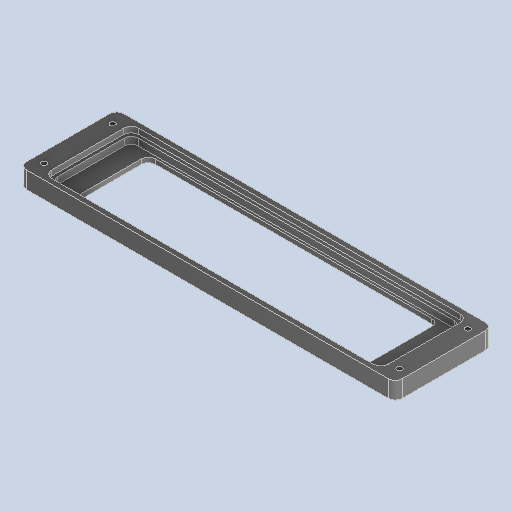
# Autodesk Inventor part: TorsoButtonCoverFrame
Saved by Autodesk Inventor 2024.2 (Build 282272000, 272)
## iProperties
Created: 2024-01-28
Part Number: TorsoButtonCoverFrame
Material: Acetal Resin, Black
Document SubType Name: Modeling
Designer: Masato Kubotera
Density: 1.425 g/cm^3
Appearance: Smooth - Black
Vendor: meviy
Mass: 8.31049 g
Surface Area: 66.1312 cm^2
Volume: 5.83192 cm^3
Author: Masato Kubotera
Autodesk Inventor part; units mm, degrees
ref_plane "YZ Plane" through (0, 0, 0) normal (1, 0, 0) x (0, 1, 0)
ref_plane "XZ Plane" through (0, 0, 0) normal (0, 1, 0) x (-1, 0, 0)
ref_plane "XY Plane" through (0, 0, 0) normal (0, 0, 1) x (1, 0, 0)
derived "TorsoUpperFrame.ipt"
sketch "Sketch1" plane through (0, 0, 0) normal (0, 0, 1) x (1, 0, 0)
  line L0 (-50, -90) -> (50, -90)
  line L1 (50, -90) -> (50, 90)
  line L2 (50, 90) -> (-50, 90)
  line L3 (-50, 90) -> (-50, -90)
  line L4 (-50, -90) -> (50, 90) construction
  line L5 (50, -90) -> (-50, 90) construction
  line L6 (-50, 0) -> (50, 0)
  line L7 (0, -90) -> (0, 90) construction
  circle A0 centre (0, 0) radius 18.75
  line L8 (-12, -16) -> (31, -16) construction
  line L9 (31, -16) -> (31, 16) construction
  line L10 (31, 16) -> (-12, 16) construction
  line L11 (-12, 16) -> (-12, -16) construction
  line L12 (-12, -16) -> (31, 16) construction
  line L13 (31, -16) -> (-12, 16) construction
  line L14 (1, -13.5) -> (28, -13.5) construction
  line L15 (28, -13.5) -> (28, 13.5) construction
  line L16 (28, 13.5) -> (1, 13.5) construction
  line L17 (1, 13.5) -> (1, -13.5) construction
  line L18 (1, -13.5) -> (28, 13.5) construction
  line L19 (28, -13.5) -> (1, 13.5) construction
  line L20 (9.61, -16.1) -> (31.1, -16.1)
  line L21 (31.1, -16.1) -> (31.1, 16.1)
  line L22 (31.1, 16.1) -> (9.61, 16.1)
  line L23 (50, 85) -> (38, 85)
  line L24 (38, 85) -> (38, 90)
  line L25 (-15, 90) -> (-15, 85)
  line L26 (-15, 85) -> (15, 85)
  line L27 (15, 85) -> (15, 90)
  arc A1 (38, 85) -> (42, 85) centre (40, 85) ccw
  arc A2 (11, 85) -> (15, 85) centre (13, 85) ccw
  arc A3 (-15, 85) -> (-11, 85) centre (-13, 85) ccw
  line L28 (-38, 85) -> (-38, 90)
  arc A4 (-42, 85) -> (-38, 85) centre (-40, 85) ccw
  line L29 (-50, 85) -> (-38, 85)
  line L30 (46, 85) -> (46, 79) construction
  line L31 (-46, 85) -> (-46, 79) construction
  circle A5 centre (0, 0) radius 29 construction
  line L32 (-41.5, 0) -> (-41.5, 53.2624)
  line L33 (-41.5, 53.2624) -> (-50, 58.1699)
  circle A6 centre (-42.5, 62.5) radius 7.5 construction
  circle A7 centre (-42.5, 62.5) radius 5 construction
  line L34 (-70, -90.6743) -> (-70, 90) construction
  line L35 (70, -90.6743) -> (70, 90) construction
  line L36 (-50, 62.5) -> (-37.5, 62.5) construction
  circle A8 centre (-42.5, -62.5) radius 5 construction
  circle A9 centre (-42.5, -62.5) radius 7.5 construction
  line L37 (-41.5, 0) -> (-41.5, -53.2624)
  line L38 (-41.5, -53.2624) -> (-50, -58.1699)
  line L39 (-50, -85) -> (-38, -85)
  line L40 (-38, -85) -> (-38, -90)
  arc A10 (-38, -85) -> (-42, -85) centre (-40, -85) ccw
  line L41 (-15, -85) -> (15, -85)
  arc A11 (-11, -85) -> (-15, -85) centre (-13, -85) ccw
  arc A12 (15, -85) -> (11, -85) centre (13, -85) ccw
  line L42 (-15, -90) -> (-15, -85)
  line L43 (15, -85) -> (15, -90)
  arc A13 (42, -85) -> (38, -85) centre (40, -85) ccw
  line L44 (38, -85) -> (38, -90)
  line L45 (50, -85) -> (38, -85)
  line L46 (-36.6858, 30.1642) -> (-36.6858, 46.0358)
  line L47 (-34.6858, 48.0358) -> (-18.8142, 48.0358)
  line L48 (-35.6, 46.95) -> (-35.6, 29.25) construction
  line L49 (-17.9, 46.95) -> (-35.6, 46.95) construction
  line L50 (-36.1, 28.75) -> (-36.1, 47.45) construction
  line L51 (-36.1, 47.45) -> (-17.4, 47.45) construction
  line L52 (-35.6, 29.25) -> (-17.9, 29.25) construction
  line L53 (-35.6, 46.95) -> (-17.9, 29.25) construction
  line L54 (-17.9, 46.95) -> (-35.6, 29.25) construction
  line L55 (-18.8142, 28.1642) -> (-34.6858, 28.1642)
  line L56 (-16.8142, 48.0358) -> (-36.6858, 28.1642) construction
  line L57 (-36.6858, 48.0358) -> (-16.8142, 28.1642) construction
  line L58 (-17.4, 28.75) -> (-36.1, 28.75) construction
  line L59 (-36.1, 47.45) -> (-17.4, 28.75) construction
  line L60 (-17.4, 47.45) -> (-36.1, 28.75) construction
  line L61 (-17.9, 29.25) -> (-17.9, 46.95) construction
  line L62 (-17.4, 47.45) -> (-17.4, 28.75) construction
  arc A14 (-18.8142, 28.1642) -> (-16.8142, 30.1642) centre (-18.8142, 30.1642) ccw
  line L63 (-16.8142, 46.0358) -> (-16.8142, 30.1642)
  arc A15 (-36.6858, 30.1642) -> (-34.6858, 28.1642) centre (-34.6858, 30.1642) ccw
  arc A16 (-16.8142, 46.0358) -> (-18.8142, 48.0358) centre (-18.8142, 46.0358) ccw
  arc A17 (-34.6858, 48.0358) -> (-36.6858, 46.0358) centre (-34.6858, 46.0358) ccw
  arc A18 (-18.8142, -48.0358) -> (-16.8142, -46.0358) centre (-18.8142, -46.0358) ccw
  line L64 (-16.8142, -46.0358) -> (-16.8142, -30.1642)
  line L65 (-17.9, -29.25) -> (-17.9, -46.95) construction
  line L66 (-17.4, -47.45) -> (-17.4, -28.75) construction
  arc A19 (-16.8142, -30.1642) -> (-18.8142, -28.1642) centre (-18.8142, -30.1642) ccw
  line L67 (-34.6858, -48.0358) -> (-18.8142, -48.0358)
  line L68 (-17.9, -46.95) -> (-35.6, -46.95) construction
  line L69 (-36.1, -47.45) -> (-17.4, -47.45) construction
  line L70 (-18.8142, -28.1642) -> (-34.6858, -28.1642)
  line L71 (-35.6, -29.25) -> (-17.9, -29.25) construction
  line L72 (-35.6, -46.95) -> (-17.9, -29.25) construction
  line L73 (-17.9, -46.95) -> (-35.6, -29.25) construction
  line L74 (-17.4, -28.75) -> (-36.1, -28.75) construction
  line L75 (-36.1, -47.45) -> (-17.4, -28.75) construction
  line L76 (-17.4, -47.45) -> (-36.1, -28.75) construction
  line L77 (-16.8142, -48.0358) -> (-36.6858, -28.1642) construction
  line L78 (-36.6858, -48.0358) -> (-16.8142, -28.1642) construction
  arc A20 (-36.6858, -46.0358) -> (-34.6858, -48.0358) centre (-34.6858, -46.0358) ccw
  line L79 (-36.6858, -30.1642) -> (-36.6858, -46.0358)
  line L80 (-35.6, -46.95) -> (-35.6, -29.25) construction
  line L81 (-36.1, -28.75) -> (-36.1, -47.45) construction
  arc A21 (-34.6858, -28.1642) -> (-36.6858, -30.1642) centre (-34.6858, -30.1642) ccw
  arc A22 (0, 16) -> (-12, 10.583) centre (0, 0) ccw construction
  arc A23 (-12, -10.583) -> (0, -16) centre (0, 0) ccw construction
  line L82 (-26.75, 38.1) -> (-26.75, -38.1) construction
  line L83 (-14.5, 55) -> (-27.6628, 55)
  arc A24 (-39.3295, 80) -> (-41.0778, 77.0287) centre (-39.3295, 78) ccw
  line L84 (-41.5, 16) -> (-37.5, 16) construction
  line L85 (-41.5, -16) -> (-37.5, -16) construction
  line L86 (-37.25, -49) -> (-16.25, -49) construction
  line L87 (-14.25, -47) -> (-14.25, 47) construction
  line L88 (-16.25, 49) -> (-37.25, 49) construction
  line L89 (-39.25, 47) -> (-39.25, -47) construction
  line L90 (-39.25, -49) -> (-14.25, 49) construction
  line L91 (-14.25, -49) -> (-39.25, 49) construction
  line L92 (-16.75, 52) -> (-36.75, 52) construction
  circle A25 centre (-16.75, 52) radius 1 construction
  circle A26 centre (-16.75, 52) radius 2 construction
  line L93 (-39, -55) -> (-14.5, -55) construction
  line L94 (-12.5, -53) -> (-12.5, 53) construction
  line L95 (-14.5, 55) -> (-39, 55) construction
  line L96 (-41, 53) -> (-41, -53) construction
  line L97 (-41, -55) -> (-12.5, 55) construction
  line L98 (-12.5, -55) -> (-41, 55) construction
  arc A27 (-12.5, 53) -> (-14.5, 55) centre (-14.5, 53) ccw construction
  arc A28 (-39, 55) -> (-41, 53) centre (-39, 53) ccw construction
  arc A29 (-41, -53) -> (-39, -55) centre (-39, -53) ccw construction
  arc A30 (-14.5, -55) -> (-12.5, -53) centre (-14.5, -53) ccw construction
  arc A31 (-37.25, 49) -> (-39.25, 47) centre (-37.25, 47) ccw construction
  arc A32 (-14.25, 47) -> (-16.25, 49) centre (-16.25, 47) ccw construction
  arc A33 (-16.25, -49) -> (-14.25, -47) centre (-16.25, -47) ccw construction
  arc A34 (-39.25, -47) -> (-37.25, -49) centre (-37.25, -47) ccw construction
  line L99 (-17.75, 22.5) -> (-35.75, 22.5) construction
  line L100 (-35.75, 22.5) -> (-35.75, -22.5) construction
  line L101 (-35.75, -22.5) -> (-17.75, -22.5) construction
  line L102 (-17.75, -22.5) -> (-17.75, 22.5) construction
  line L103 (-17.75, 22.5) -> (-35.75, -22.5) construction
  line L104 (-35.75, 22.5) -> (-17.75, -22.5) construction
  line L105 (41.0778, 77.0287) -> (13.0754, 26.6244)
  line L106 (15.6978, 25.1674) -> (43.2517, 74.7643)
  line L107 (47, 73.7931) -> (47, 3.5)
  line L108 (29.1, 18.1) -> (17.9933, 18.1)
  arc A35 (47, 73.7931) -> (43.2517, 74.7643) centre (45, 73.7931) ccw
  line L109 (-36.6858, 23.1642) -> (-36.6858, 0)
  line L110 (-34.37, -22.5) -> (-34.37, 22.5) construction
  line L111 (-29.25, 5.12) -> (-24.25, 5.12) construction
  line L112 (-24.25, 5.12) -> (-24.25, 10.12) construction
  line L113 (-24.25, 10.12) -> (-29.25, 10.12) construction
  line L114 (-29.25, 10.12) -> (-29.25, 5.12) construction
  line L115 (-29.25, 5.12) -> (-24.25, 10.12) construction
  line L116 (-24.25, 5.12) -> (-29.25, 10.12) construction
  circle A36 centre (-26.75, 7.62) radius 1.5 construction
  line L117 (-32.99, -22.5) -> (-32.99, 22.5) construction
  line L118 (-29.25, 25.36) -> (-29.25, 20.36) construction
  line L119 (-29.25, 20.36) -> (-24.25, 20.36) construction
  line L120 (-24.25, 20.36) -> (-24.25, 25.36) construction
  circle A37 centre (-26.75, 22.86) radius 1.5 construction
  line L121 (-24.25, 25.36) -> (-29.25, 25.36) construction
  arc A38 (-23.5471, 4.0762) -> (-29, 0) centre (-24.75, 0) ccw
  arc A39 (-23.5471, 4.0762) -> (-21.0458, 5.4896) centre (-22.9811, 5.9944) ccw
  arc A40 (5.7687, 20.971) -> (8.2434, 22.4305) centre (6.2992, 22.8994) ccw
  line L122 (-12.5, 27.3962) -> (-12.5, 53)
  arc A41 (-8.2434, 22.4305) -> (-5.7687, 20.971) centre (-6.2992, 22.8994) ccw
  arc A42 (-12.5, 27.3962) -> (-11.1, 25.4884) centre (-10.5, 27.3962) ccw
  line L123 (-39.3295, 80) -> (39.3295, 80)
  arc A43 (41.0778, 77.0287) -> (39.3295, 80) centre (39.3295, 78) ccw
  line L124 (45, 1.5) -> (35.1, 1.5)
  line L125 (33.1, 3.5) -> (33.1, 14.1)
  arc A44 (45, 1.5) -> (47, 3.5) centre (45, 3.5) ccw
  arc A45 (33.1, 3.5) -> (35.1, 1.5) centre (35.1, 3.5) ccw
  arc A46 (33.1, 14.1) -> (29.1, 18.1) centre (29.1, 14.1) ccw
  line L126 (-41.0778, 77.0287) -> (-29.4111, 56.0287)
  arc A47 (15.6978, 25.1674) -> (15.6898, 23.2395) centre (17.4462, 24.1961) ccw
  arc A48 (16.0474, 20.5621) -> (17.9933, 18.1) centre (17.9933, 20.1) ccw
  arc A49 (-17.2299, 13.2738) -> (-21.0458, 5.4896) centre (0, 0) ccw
  arc A50 (5.7687, 20.971) -> (-5.7687, 20.971) centre (0, 0) ccw
  arc A51 (11.6624, 25.624) -> (13.0754, 26.6244) centre (11.3271, 27.5956) ccw
  arc A52 (15.6978, 25.1674) -> (15.4533, 24.3645) centre (17.4462, 24.1961) ccw
  arc A53 (11.6624, 25.624) -> (8.2434, 22.4305) centre (12.375, 21.4341) ccw
  arc A54 (-8.2434, 22.4305) -> (-11.1, 25.4884) centre (-12.375, 21.4341) ccw
  arc A55 (16.0474, 20.5621) -> (15.6898, 23.2395) centre (12.375, 21.4341) ccw
  arc A56 (-29.4111, 56.0287) -> (-27.6628, 55) centre (-27.6628, 57) ccw
  line L127 (-36.6858, 23.1642) -> (-36.6858, 30.1642)
  line L128 (-16.8142, 30.1642) -> (-16.8142, 14.4944)
  arc A57 (-17.2299, 13.2738) -> (-16.8142, 14.4944) centre (-18.8142, 14.4944) ccw
  circle A58 centre (0, 64) radius 7.5
  point P0 (9.5, 0)
  point P1 (14.5, 0)
  point P2 (24.75, 0)
  point P3 (-12.375, 21.4341)
  point P4 (-12.375, -21.4341)
  point P5 (12.375, -21.4341)
  point P6 (-37.5, -62.5)
  point P7 (-46, -85)
  point P8 (46, -85)
  point P9 (50, 69.4499)
  point P10 (50, 77.5499)
  point P11 (-46, -79)
  point P12 (-26.75, 38.1)
  point P13 (-26.75, 38.1)
  point P14 (-26.75, -38.1)
  point P15 (-26.75, 38.1)
  point P16 (-35, 55)
  point P17 (-28.8396, 55)
  point P18 (-26.75, 0)
  point P19 (-16.75, -52)
  point P20 (-36.75, -52)
  point P21 (43.8396, 82)
  point P22 (42.2091, 72.8876)
  point P23 (47, 72.8875)
  point P24 (47, 1.5)
  point P25 (33.1, 18.1)
  point P26 (-12.5, 51.9999)
  point P27 (40, 83)
  point P28 (-16.8142, 24.516)
  point P29 (-16.8142, 13.7965)
sketch "Sketch2" plane through (0, 0, 0) normal (0, 0, 1) x (1, 0, 0)
  line L0 (-41, 53) -> (-41, -53) projected
  arc A0 (-41, -53) -> (-39, -55) centre (-39, -53) ccw projected
  line L1 (-39, -55) -> (-14.5, -55) projected
  arc A1 (-14.5, -55) -> (-12.5, -53) centre (-14.5, -53) ccw projected
  line L2 (-12.5, -53) -> (-12.5, 53) projected
  arc A2 (-12.5, 53) -> (-14.5, 55) centre (-14.5, 53) ccw projected
  line L3 (-14.5, 55) -> (-39, 55) projected
  arc A3 (-39, 55) -> (-41, 53) centre (-39, 53) ccw projected
  line L4 (-16.25, 49.25) -> (-37.25, 49.25)
  line L5 (-39.5, 47) -> (-39.5, -47)
  line L6 (-37.25, -49.25) -> (-16.25, -49.25)
  line L7 (-14, -47) -> (-14, 47)
  line L8 (-14, 49.25) -> (-39.5, -49.25) construction
  line L9 (-39.5, 49.25) -> (-14, -49.25) construction
  line L10 (-16.25, 49) -> (-37.25, 49) construction
  arc A4 (-14.25, 47) -> (-16.25, 49) centre (-16.25, 47) ccw construction
  line L11 (-14.25, -47) -> (-14.25, 47) construction
  arc A5 (-16.25, -49) -> (-14.25, -47) centre (-16.25, -47) ccw construction
  line L12 (-37.25, -49) -> (-16.25, -49) construction
  arc A6 (-39.25, -47) -> (-37.25, -49) centre (-37.25, -47) ccw construction
  line L13 (-39.25, 47) -> (-39.25, -47) construction
  arc A7 (-37.25, 49) -> (-39.25, 47) centre (-37.25, 47) ccw construction
  arc A8 (-16.25, -49.25) -> (-14, -47) centre (-16.25, -47) ccw
  arc A9 (-14, 47) -> (-16.25, 49.25) centre (-16.25, 47) ccw
  arc A10 (-37.25, 49.25) -> (-39.5, 47) centre (-37.25, 47) ccw
  arc A11 (-39.5, -47) -> (-37.25, -49.25) centre (-37.25, -47) ccw
  line L14 (-36.5, -48.25) -> (-17, -48.25)
  line L15 (-15, -46.25) -> (-15, 46.25)
  line L16 (-17, 48.25) -> (-36.5, 48.25)
  line L17 (-38.5, 46.25) -> (-38.5, -46.25)
  line L18 (-38.5, -48.25) -> (-15, 48.25) construction
  line L19 (-15, -48.25) -> (-38.5, 48.25) construction
  arc A12 (-15, 46.25) -> (-17, 48.25) centre (-17, 46.25) ccw
  arc A13 (-36.5, 48.25) -> (-38.5, 46.25) centre (-36.5, 46.25) ccw
  arc A14 (-38.5, -46.25) -> (-36.5, -48.25) centre (-36.5, -46.25) ccw
  arc A15 (-17, -48.25) -> (-15, -46.25) centre (-17, -46.25) ccw
  line L20 (-35.75, 42.5) -> (-17.75, 42.5)
  line L21 (-15.75, 40.5) -> (-15.75, -40.5)
  line L22 (-17.75, -42.5) -> (-35.75, -42.5)
  line L23 (-37.75, -40.5) -> (-37.75, 40.5)
  line L24 (-37.75, 42.5) -> (-15.75, -42.5) construction
  line L25 (-15.75, 42.5) -> (-37.75, -42.5) construction
  line L26 (-35.75, -22.5) -> (-17.75, -22.5) construction
  line L27 (-17.75, -22.5) -> (-17.75, 22.5) construction
  line L28 (-35.75, 22.5) -> (-35.75, -22.5) construction
  line L29 (-17.75, 22.5) -> (-35.75, 22.5) construction
  arc A16 (-15.75, 40.5) -> (-17.75, 42.5) centre (-17.75, 40.5) ccw
  arc A17 (-35.75, 42.5) -> (-37.75, 40.5) centre (-35.75, 40.5) ccw
  arc A18 (-17.75, -42.5) -> (-15.75, -40.5) centre (-17.75, -40.5) ccw
  arc A19 (-37.75, -40.5) -> (-35.75, -42.5) centre (-35.75, -40.5) ccw
  point P0 (0, 0)
  point P1 (-36.75, 52)
  point P2 (-16.75, 52)
  point P3 (-16.75, -52)
  point P4 (-36.75, -52)
  point P5 (-26.75, 0)
  point P6 (-26.75, 0)
  dimension "d4" = 0.25
  dimension "d5" = 0.25
  dimension "d6" = 2
  dimension "d7" = 2.25
  dimension "d9" = 2
  dimension "d10" = 1
  dimension "d11" = 1
  dimension "d26" = 2
  dimension "d27" = 2
  dimension "d31" = 20
  constraints: 36 end point, 24 point on circle, 24 point on line, 24 tangent, 12 centre point, 9 equal radius, 6 midpoint, 6 parallel, 3 horizontal, 3 perpendicular, 1 coincident
  measures "d4" distance between parallel lines of L7 L11
  measures "d5" distance between parallel lines of L4 L10
  measures "d6" radius of A4
  measures "d7" radius of A9
  measures "d9" radius of A13
  measures "d10" distance between parallel lines of L15 L7
  measures "d11" distance between parallel lines of L4 L16
  measures "d26" radius of A16
  measures "d27" distance between parallel lines of L21 L27
  measures "d31" distance between parallel lines of L20 L29
extrude "Extrusion1" add sketch "Sketch2" against normal blind 5 contours A3 L3 A2 L2 A1 L1 A0 L0 | A9 L7 A8 L6 A11 L5 A10 L4 | A14 L17 A13 L16 A12 L15 A15 L14 | L20 A16 L21 A18 L22 A19 L23 A17
extrude "Extrusion2" cut sketch "Sketch2" against normal blind 1.6 contours A9 L7 A8 L6 A11 L5 A10 L4
extrude "Extrusion3" cut sketch "Sketch2" against normal blind 3.6 contours A14 L17 A13 L16 A12 L15 A15 L14 | L20 A16 L21 A18 L22 A19 L23 A17
hole "Hole1" at (-36.75, 52, 0) at (-16.75, 52, 0) at (-16.75, -52, 0) at (-36.75, -52, 0) direction (0, 0, -1) diameter 1.567 end through all thread size "M2x0.4" class "6H" standard "ANSI Metric M Profile"
extrude "Extrusion4" cut sketch "Sketch2" against normal through all contours L20 A16 L21 A18 L22 A19 L23 A17
equation "\"d5\" = d4"
equation "\"d7\" = d6 + d4"
equation "\"d11\" = d10"
body "Solid1"
